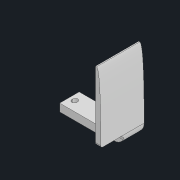
# Autodesk Inventor part: base49
Saved by Autodesk Inventor 2022 (Build 260153000, 153)
## iProperties
Created: 2021-10-06
Part Number: base49
Material: 一般
Document SubType Name: Modeling
Designer: Yuta Kage
Density: 1 g/cm^3
Appearance: 既定
Author: Yuta Kage
Autodesk Inventor part; units mm, degrees
ref_plane "YZ Plane" through (0, 0, 0) normal (1, 0, 0) x (0, 1, 0)
ref_plane "XZ Plane" through (0, 0, 0) normal (0, 1, 0) x (-1, 0, 0)
ref_plane "XY Plane" through (0, 0, 0) normal (0, 0, 1) x (1, 0, 0)
sketch "スケッチ1" plane through (0, 0, 0) normal (0, 0, 1) x (1, 0, 0)
  line L0 (0, 0) -> (0, 5)
  line L1 (0, 5) -> (50, 5)
  line L2 (55, 10) -> (55, 73)
  line L3 (55, 73) -> (60, 73)
  line L4 (60, 73) -> (60, 10)
  line L5 (50, 0) -> (0, 0)
  arc A0 (50, 0) -> (60, 10) centre (50, 10) ccw
  line L6 (0, 0) -> (50, 0)
  line L7 (40, 0) -> (40, -2)
  line L8 (40, -2) -> (0, -2)
  line L9 (0, -2) -> (0, 0)
  arc A1 (50, 5) -> (55, 10) centre (50, 10) ccw
  point P0 (60, 0)
  point P1 (55, 5)
  point P2 (40, 0)
  dimension "d0" = 55
  dimension "d1" = 73
  dimension "d2" = 5
  dimension "d3" = 5
  dimension "d5" = 10
  dimension "d34" = 2
  dimension "d35" = 40
  dimension "d58" = 5
  constraints: 20 end point, 6 perpendicular, 6 point on line, 4 point on circle, 4 tangent, 2 centre point, 2 parallel, 1 horizontal, 1 vertical
  measures "d0" distance of point (55, 5) L0.end
  measures "d1" distance of L3.end point (60, 0)
  measures "d2" distance of L2.end L3.end
  measures "d3" distance of L0.start L0.end
  measures "d5" radius of A0
  measures "d34" distance of L7.start L7.end
  measures "d35" distance of L7.end L8.end
  measures "d58" radius of A1
extrude "押し出し1" add sketch "スケッチ1" along normal mid plane 18
sketch "スケッチ2" plane through (0, 5, 9) normal (0, 1, 0) x (1, 0, 0)
  line L0 (50, 0) -> (0, 0) projected
  line L1 (0, 18) -> (0, 0) projected
  point P0 (5, 9)
  point P1 (35, 9)
  dimension "d8" = 30
  dimension "d59" = 9
  dimension "d60" = 5
  constraints: 1 horizontal alignment
  measures "d8" distance of point (5, 9) point (35, 9)
  measures "d59" distance from line of L0 point (5, 9)
  measures "d60" distance from line of L1 point (5, 9)
hole "穴1" at (5, 5, 0) at (35, 5, 0) direction (0, -1, 0) diameter 4.5 end through all clearance for "Flat Head Machine Screw" size "M4" standard "Ansi Metric M Profile"
sketch "スケッチ3" plane through (0, 0, 9) normal (0, 0, 1) x (1, 0, 0)
  line L0 (60, 10) -> (60, 73) projected
  line L1 (60, 73) -> (55, 73) projected
  line L2 (55, 73) -> (55, 10) projected
  line L3 (50, 5) -> (0, 5) projected
  line L4 (0, 5) -> (0, -2) projected
  arc A0 (50, 0) -> (60, 10) centre (50, 10) ccw projected
  line L5 (0, -2) -> (40, -2) projected
  line L6 (40, -2) -> (40, 0) projected
  line L7 (40, 0) -> (50, 0) projected
  line L8 (60, 10) -> (55, 10)
  line L9 (55, 73) -> (55, 10) projected
  arc A1 (50, 5) -> (55, 10) centre (50, 10) ccw projected
  point P0 (55, 6)
  point P1 (55, 10)
  constraints: 3 end point, 1 perpendicular
extrude "押し出し2" add sketch "スケッチ3" along normal blind 22 contours L8 L2 L1 L0
sketch "スケッチ4" plane through (0, -2, 9) normal (0, -1, 0) x (1, 0, 0)
  line L0 (0, -18) -> (40, -18)
  line L1 (40, -18) -> (40, -14.653)
  line L2 (40, -14.653) -> (0, -14.653)
  line L3 (0, -14.653) -> (0, -18)
  point P0 (0, -9)
  dimension "d20" = 40
  dimension "d21" = 3.347
  constraints: 8 end point, 2 parallel, 1 coincident, 1 horizontal, 1 perpendicular
  measures "d20" distance of L0.start L0.end
  measures "d21" distance of L0.end L1.end
extrude "押し出し3" add sketch "スケッチ4" along normal blind 8
chamfer "面取り1" distance 0.5 angle 45 1 edges at (20, -2, -5.653)
sketch "スケッチ6" plane through (0, 5, -9) normal (0, 1, 0) x (1, 0, 0)
  circle A0 centre (5, -9) radius 2.25 projected
  circle A1 centre (35, -9) radius 2.25 projected
  line L0 (5, -9.5) -> (5, -8.5) construction
  line L1 (7.25, -9.5) -> (7.25, -8.5)
  line L2 (2.75, -8.5) -> (2.75, -9.5)
  arc A2 (2.75, -9.5) -> (7.25, -9.5) centre (5, -9.5) ccw
  arc A3 (7.25, -8.5) -> (2.75, -8.5) centre (5, -8.5) ccw
  line L3 (35, -9.5) -> (35, -8.5) construction
  line L4 (32.75, -9.5) -> (32.75, -8.5)
  line L5 (37.25, -8.5) -> (37.25, -9.5)
  arc A4 (32.75, -9.5) -> (37.25, -9.5) centre (35, -9.5) ccw
  arc A5 (37.25, -8.5) -> (32.75, -8.5) centre (35, -8.5) ccw
  point P0 (0, -9)
  dimension "d37" = 1
  dimension "d38" = 1
  constraints: 16 end point, 10 tangent, 8 point on circle, 4 centre point, 3 parallel, 2 midpoint, 1 vertical
  measures "d37" distance of L2.start L2.end
  measures "d38" distance of L4.start L4.end
extrude "押し出し5" cut sketch "スケッチ6" against normal blind 18
sketch "スケッチ5" plane through (0, 0, 31) normal (0, 0, 1) x (1, 0, 0)
  line L0 (55, 73) -> (60, 73) projected
  line L1 (60, 73) -> (60, 10) projected
  line L2 (55, 73) -> (55, 10) projected
  line L3 (60, 10) -> (60, 73) construction
  line L4 (60, 73) -> (56, 73) construction
  spline S0 degree 2 poles (60, 10) (60, 73) (56, 73) knots 1 1 1 2 2 2
  line L5 (60, 73) -> (55, 73) projected
  point P0 (0, 0)
  point P1 (55, 13)
  point P2 (55, 8)
  dimension "d30" = 1
  constraints: 1 coincident, 1 point on line, 3 other
  measures "d30" distance of L0.start L4.end
extrude "押し出し4" cut sketch "スケッチ5" against normal through all
fillet "フィレット10" radius 2 1 edges at (57.5, 10, 31)
fillet "フィレット11" radius 5 1 edges at (57.5, 10, 9)
